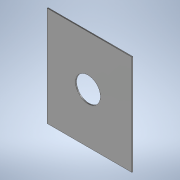
# Autodesk Inventor part: Placa gatilho
Saved by Autodesk Inventor 2021 (Build 250183000, 183)
## iProperties
Created: 2020-12-03
Part Number: Placa gatilho
Material: Liga de Nickel-Copper 400
Document SubType Name: Modeling
Designer: Lucas Moura
Density: 8.83 g/cm^3
Appearance: Cromado - Preto polido
Author: Lucas Moura
Autodesk Inventor part; units mm, degrees
ref_plane "YZ Plane" through (0, 0, 0) normal (1, 0, 0) x (0, 1, 0)
ref_plane "XZ Plane" through (0, 0, 0) normal (0, 1, 0) x (-1, 0, 0)
ref_plane "XY Plane" through (0, 0, 0) normal (0, 0, 1) x (1, 0, 0)
sketch "Sketch1" plane through (0, 0, 0) normal (0, 0, 1) x (1, 0, 0)
  line L0 (0, 0) -> (1.7, 0)
  line L1 (1.7, 0) -> (1.7, 2)
  line L2 (1.7, 2) -> (0, 2)
  line L3 (0, 2) -> (0, 0)
  dimension "d0" = 2
  dimension "d1" = 1.7
  constraints: 8 end point, 2 parallel, 1 horizontal, 1 perpendicular
  measures "d0" distance of L2.end L0.start
  measures "d1" distance of L1.end L2.end
extrude "Extrusion1" add sketch "Sketch1" along normal blind 0.02
sketch "Sketch2" plane through (0, 0, 0.02) normal (0, 0, 1) x (1, 0, 0)
  line L0 (0, 2) -> (0, 0) projected
  line L1 (0, 2) -> (1.64, 2)
  line L2 (1.64, 2) -> (1.64, 0)
  line L3 (0, 0) -> (0, 2)
  circle A0 centre (0.82, 1) radius 0.25
  line L4 (0, 0) -> (1.64, 0)
  dimension "d9" = 0.5
  dimension "d10" = 1.64
  dimension "d11" = 2
  constraints: 8 end point, 2 horizontal, 1 centre point, 1 parallel, 1 perpendicular
  measures "d9" diameter of A0
  measures "d10" distance of L3.start L2.end
  measures "d11" distance of L1.end L2.end
extrude "Extrusion2" cut sketch "Sketch2" against normal through all contours A0
body "Solid1"
